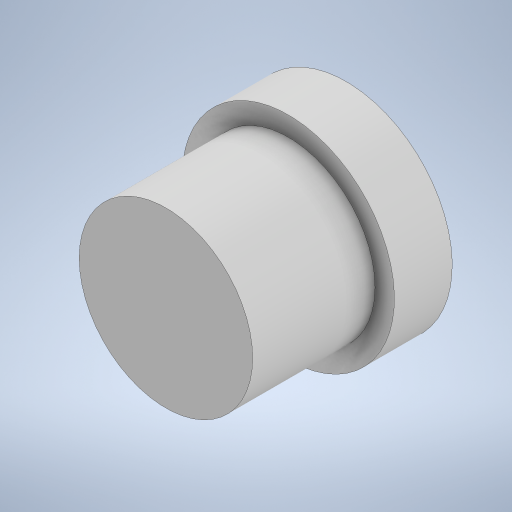
# Autodesk Inventor part: att_pin
Saved by Autodesk Inventor 2023.1 (Build 271208000, 208)
## iProperties
Created: 2024-12-03
Part Number: att_pin
Material: Типовые
Document SubType Name: Modeling
Designer: DELL
Density: 1 g/cm^3
Appearance: По умолчанию
Author: DELL
Autodesk Inventor part; units mm, degrees
(part 1 of 2)
ref_plane "YZ Plane" through (0, 0, 0) normal (1, 0, 0) x (0, 1, 0)
ref_plane "XZ Plane" through (0, 0, 0) normal (0, 1, 0) x (-1, 0, 0)
ref_plane "XY Plane" through (0, 0, 0) normal (0, 0, 1) x (1, 0, 0)
sketch "Эскиз1" plane through (0, 0, 0) normal (0, 0, 1) x (1, 0, 0)
  circle A0 centre (5.7181, 0.7273) radius 3.0026 construction
  ellipse E0 centre (5.709, 0.7156) end of major axis (2.2813, -3.5903) minor radius 5.5036 projected
  circle A1 centre (5.709, 0.7156) radius 2.75
  point P0 (0, 0)
  dimension "d4" = 5.5
  constraints: 1 centre point, 1 coincident, 1 other
  measures "d4" diameter of A1
extrude "Выдавливание1" add sketch "Эскиз1" along normal blind 3
sketch "Эскиз2" plane through (0, 0, 3) normal (0, 0, 1) x (1, 0, 0)
  spline S0 degree 3 poles (20.6934, -4.2961) (20.668, -4.2959) (20.6158, -4.2949) (20.5384, -4.2922) (20.4629, -4.2881) (20.3923, -4.2832) (20.3162, -4.2759) (20.2564, -4.2711) (20.212, -4.2637) (20.1912, -4.2611) (20.1707, -4.2589) (20.1505, -4.2572) (20.1304, -4.2562) (20.1104, -4.2558) (20.0904, -4.256) (20.0703, -4.2569) (20.0501, -4.2587) (20.0294, -4.2614) (20.0083, -4.2652) (19.9866, -4.2704) (19.964, -4.2773) (19.9404, -4.2862) (19.9158, -4.2978) (19.8904, -4.3128) (19.8644, -4.3319) (19.8387, -4.3557) (19.8146, -4.3847) (19.7945, -4.417) (19.7684, -4.4768) (19.7397, -4.5638) (19.7039, -4.6481) (19.6841, -4.7103) (19.6779, -4.7478) (19.6769, -4.7855) (19.6805, -4.8204) (19.6874, -4.8518) (19.6967, -4.8799) (19.7075, -4.9048) (19.7193, -4.9271) (19.7318, -4.9471) (19.7447, -4.9654) (19.7581, -4.9822) (19.7718, -4.9978) (19.7858, -5.0125) (19.8003, -5.0265) (19.8152, -5.0398) (19.8305, -5.0527) (19.8463, -5.0651) (19.8626, -5.0773) (19.8794, -5.0892) (19.8968, -5.1009) (19.9351, -5.1246) (19.9832, -5.1604) (20.0452, -5.2051) (20.1015, -5.248) (20.1609, -5.2947) (20.2209, -5.3437) (20.2608, -5.3774) (20.2801, -5.394) knots -0.738433 -0.738433 -0.738433 -0.738433 -0.721428 -0.703497 -0.686646 -0.670877 -0.656188 -0.635555 -0.630797 -0.626128 -0.621536 -0.617009 -0.612531 -0.608082 -0.603638 -0.599173 -0.594654 -0.590038 -0.585279 -0.580318 -0.575085 -0.569501 -0.563479 -0.55693 -0.549778 -0.541982 -0.533567 -0.524647 -0.516621 -0.490028 -0.463434 -0.455408 -0.446488 -0.438073 -0.430277 -0.423125 -0.416576 -0.410554 -0.40497 -0.399737 -0.394776 -0.390017 -0.385402 -0.380882 -0.376417 -0.371974 -0.367524 -0.363046 -0.358519 -0.353927 -0.349258 -0.3445 -0.323867 -0.309178 -0.293409 -0.276558 -0.258627 -0.241622 -0.241622 -0.241622 -0.241622 projected
  arc A0 (20.6934, -4.2961) -> (21.0569, -3.0396) centre (5.7104, 0.7186) ccw projected
  spline S1 degree 3 poles (21.2935, -1.8905) (21.2683, -1.8942) (21.2165, -1.9015) (21.1397, -1.9109) (21.0645, -1.9187) (20.994, -1.9249) (20.9177, -1.9295) (20.8579, -1.9342) (20.8129, -1.9338) (20.792, -1.9344) (20.7714, -1.9355) (20.7511, -1.937) (20.7311, -1.9392) (20.7112, -1.9419) (20.6915, -1.9452) (20.6719, -1.9493) (20.6521, -1.9542) (20.6322, -1.9601) (20.612, -1.9672) (20.5913, -1.9757) (20.57, -1.986) (20.5481, -1.9985) (20.5257, -2.0139) (20.5029, -2.0326) (20.4802, -2.0555) (20.4586, -2.0831) (20.4393, -2.1155) (20.4245, -2.1505) (20.408, -2.2137) (20.3933, -2.3041) (20.3711, -2.393) (20.3613, -2.4574) (20.361, -2.4955) (20.366, -2.5329) (20.375, -2.5668) (20.3867, -2.5967) (20.4003, -2.623) (20.4149, -2.6459) (20.43, -2.6661) (20.4455, -2.6839) (20.4611, -2.6999) (20.4769, -2.7144) (20.4929, -2.7277) (20.5091, -2.7401) (20.5255, -2.7516) (20.5423, -2.7624) (20.5595, -2.7727) (20.577, -2.7826) (20.595, -2.792) (20.6135, -2.8011) (20.6325, -2.81) (20.674, -2.8274) (20.7271, -2.8553) (20.7953, -2.8897) (20.8577, -2.9233) (20.9237, -2.9601) (20.9906, -2.9991) (21.0353, -3.0262) (21.0569, -3.0396) knots -0.738433 -0.738433 -0.738433 -0.738433 -0.721428 -0.703497 -0.686646 -0.670877 -0.656188 -0.635555 -0.630797 -0.626128 -0.621536 -0.617009 -0.612531 -0.608082 -0.603638 -0.599173 -0.594654 -0.590038 -0.585279 -0.580318 -0.575085 -0.569501 -0.563479 -0.55693 -0.549778 -0.541982 -0.533567 -0.524647 -0.516621 -0.490028 -0.463434 -0.455408 -0.446488 -0.438073 -0.430277 -0.423125 -0.416576 -0.410554 -0.40497 -0.399737 -0.394776 -0.390017 -0.385402 -0.380882 -0.376417 -0.371974 -0.367524 -0.363046 -0.358519 -0.353927 -0.349258 -0.3445 -0.323867 -0.309178 -0.293409 -0.276558 -0.258627 -0.241622 -0.241622 -0.241622 -0.241622 projected
  arc A1 (21.2935, -1.8905) -> (21.4559, -0.5926) centre (5.7104, 0.7186) ccw projected
  spline S2 degree 3 poles (21.5098, 0.5793) (21.4855, 0.5717) (21.4355, 0.5565) (21.3611, 0.5352) (21.288, 0.5157) (21.2193, 0.4986) (21.1448, 0.482) (21.0864, 0.4681) (21.0419, 0.4614) (21.0213, 0.4575) (21.0011, 0.4533) (20.9813, 0.4485) (20.9619, 0.4433) (20.9428, 0.4375) (20.9238, 0.4312) (20.905, 0.424) (20.8863, 0.4161) (20.8675, 0.4072) (20.8486, 0.397) (20.8295, 0.3853) (20.8102, 0.3719) (20.7905, 0.356) (20.7707, 0.3374) (20.7511, 0.3153) (20.7323, 0.2891) (20.7153, 0.2585) (20.7013, 0.2235) (20.6921, 0.1866) (20.6858, 0.1217) (20.6854, 0.03) (20.6774, -0.0612) (20.6777, -0.1264) (20.6835, -0.1641) (20.6942, -0.2002) (20.7084, -0.2323) (20.7247, -0.26) (20.7422, -0.2838) (20.7602, -0.3042) (20.7783, -0.3218) (20.7963, -0.337) (20.8143, -0.3503) (20.8322, -0.3622) (20.85, -0.3728) (20.8679, -0.3824) (20.886, -0.3912) (20.9043, -0.3994) (20.9228, -0.4069) (20.9417, -0.4138) (20.961, -0.4204) (20.9807, -0.4264) (21.0008, -0.4322) (21.0445, -0.4429) (21.1013, -0.4622) (21.1741, -0.4855) (21.2409, -0.5089) (21.3118, -0.5349) (21.384, -0.563) (21.4324, -0.5828) (21.4559, -0.5926) knots -0.738433 -0.738433 -0.738433 -0.738433 -0.721428 -0.703497 -0.686646 -0.670877 -0.656188 -0.635555 -0.630797 -0.626128 -0.621536 -0.617009 -0.612531 -0.608082 -0.603638 -0.599173 -0.594654 -0.590038 -0.585279 -0.580318 -0.575085 -0.569501 -0.563479 -0.55693 -0.549778 -0.541982 -0.533567 -0.524647 -0.516621 -0.490028 -0.463434 -0.455408 -0.446488 -0.438073 -0.430277 -0.423125 -0.416576 -0.410554 -0.40497 -0.399737 -0.394776 -0.390017 -0.385402 -0.380882 -0.376417 -0.371974 -0.367524 -0.363046 -0.358519 -0.353927 -0.349258 -0.3445 -0.323867 -0.309178 -0.293409 -0.276558 -0.258627 -0.241622 -0.241622 -0.241622 -0.241622 projected
  arc A2 (21.5098, 0.5793) -> (21.4671, 1.8867) centre (5.7104, 0.7186) ccw projected
  spline S3 degree 3 poles (21.337, 3.0526) (21.3143, 3.0413) (21.2673, 3.0184) (21.1971, 2.9857) (21.128, 2.9551) (21.0628, 2.9274) (20.9917, 2.8994) (20.9363, 2.8765) (20.8934, 2.8629) (20.8737, 2.8559) (20.8544, 2.8485) (20.8356, 2.8408) (20.8172, 2.8326) (20.7992, 2.8239) (20.7815, 2.8146) (20.764, 2.8046) (20.7468, 2.7939) (20.7297, 2.7821) (20.7126, 2.7691) (20.6955, 2.7546) (20.6785, 2.7382) (20.6616, 2.7196) (20.645, 2.6981) (20.6291, 2.6732) (20.6146, 2.6444) (20.6025, 2.6115) (20.5942, 2.5747) (20.5909, 2.5368) (20.5948, 2.4717) (20.6088, 2.3811) (20.6151, 2.2897) (20.6257, 2.2254) (20.6372, 2.1891) (20.6534, 2.1551) (20.6725, 2.1256) (20.6929, 2.1008) (20.7139, 2.08) (20.7349, 2.0627) (20.7555, 2.0482) (20.7757, 2.036) (20.7956, 2.0256) (20.8151, 2.0167) (20.8344, 2.009) (20.8536, 2.0023) (20.8728, 1.9964) (20.8921, 1.9913) (20.9116, 1.9867) (20.9313, 1.9828) (20.9514, 1.9794) (20.9718, 1.9765) (20.9926, 1.9739) (21.0374, 1.9702) (21.0966, 1.96) (21.1721, 1.9484) (21.2417, 1.9358) (21.3159, 1.9211) (21.3916, 1.9047) (21.4424, 1.8927) (21.4671, 1.8867) knots -0.738433 -0.738433 -0.738433 -0.738433 -0.721428 -0.703497 -0.686646 -0.670877 -0.656188 -0.635555 -0.630797 -0.626128 -0.621536 -0.617009 -0.612531 -0.608082 -0.603638 -0.599173 -0.594654 -0.590038 -0.585279 -0.580318 -0.575085 -0.569501 -0.563479 -0.55693 -0.549778 -0.541982 -0.533567 -0.524647 -0.516621 -0.490028 -0.463434 -0.455408 -0.446488 -0.438073 -0.430277 -0.423125 -0.416576 -0.410554 -0.40497 -0.399737 -0.394776 -0.390017 -0.385402 -0.380882 -0.376417 -0.371974 -0.367524 -0.363046 -0.358519 -0.353927 -0.349258 -0.3445 -0.323867 -0.309178 -0.293409 -0.276558 -0.258627 -0.241622 -0.241622 -0.241622 -0.241622 projected
  arc A3 (21.337, 3.0526) -> (21.0904, 4.3372) centre (5.7104, 0.7186) ccw projected
  spline S4 degree 3 poles (20.7795, 5.4684) (20.7588, 5.4537) (20.716, 5.4238) (20.6517, 5.3805) (20.5883, 5.3394) (20.5283, 5.3019) (20.4625, 5.2631) (20.4113, 5.2318) (20.371, 5.2117) (20.3526, 5.2016) (20.3347, 5.1913) (20.3174, 5.1807) (20.3005, 5.1698) (20.2841, 5.1584) (20.2681, 5.1464) (20.2524, 5.1339) (20.237, 5.1205) (20.2219, 5.1062) (20.2071, 5.0907) (20.1925, 5.0737) (20.1783, 5.0549) (20.1645, 5.0338) (20.1514, 5.01) (20.1396, 4.9829) (20.1298, 4.9522) (20.1231, 4.9178) (20.1206, 4.8802) (20.1233, 4.8422) (20.1373, 4.7785) (20.1653, 4.6913) (20.1858, 4.602) (20.2063, 4.5401) (20.2234, 4.506) (20.2448, 4.475) (20.2682, 4.4489) (20.2923, 4.4275) (20.3163, 4.4103) (20.3397, 4.3965) (20.3623, 4.3854) (20.3842, 4.3765) (20.4054, 4.3693) (20.426, 4.3636) (20.4463, 4.359) (20.4663, 4.3554) (20.4862, 4.3526) (20.5061, 4.3505) (20.5261, 4.3491) (20.5462, 4.3483) (20.5665, 4.3481) (20.5871, 4.3484) (20.6081, 4.3491) (20.6529, 4.3524) (20.7129, 4.3517) (20.7893, 4.352) (20.8601, 4.3504) (20.9356, 4.3475) (21.013, 4.3431) (21.0651, 4.3393) (21.0904, 4.3372) knots -0.738433 -0.738433 -0.738433 -0.738433 -0.721428 -0.703497 -0.686646 -0.670877 -0.656188 -0.635555 -0.630797 -0.626128 -0.621536 -0.617009 -0.612531 -0.608082 -0.603638 -0.599173 -0.594654 -0.590038 -0.585279 -0.580318 -0.575085 -0.569501 -0.563479 -0.55693 -0.549778 -0.541982 -0.533567 -0.524647 -0.516621 -0.490028 -0.463434 -0.455408 -0.446488 -0.438073 -0.430277 -0.423125 -0.416576 -0.410554 -0.40497 -0.399737 -0.394776 -0.390017 -0.385402 -0.380882 -0.376417 -0.371974 -0.367524 -0.363046 -0.358519 -0.353927 -0.349258 -0.3445 -0.323867 -0.309178 -0.293409 -0.276558 -0.258627 -0.241622 -0.241622 -0.241622 -0.241622 projected
  arc A4 (20.7795, 5.4684) -> (20.335, 6.6987) centre (5.7104, 0.7186) ccw projected
  spline S5 degree 3 poles (19.851, 7.7673) (19.8328, 7.7495) (19.7952, 7.7132) (19.7385, 7.6604) (19.6823, 7.6099) (19.6289, 7.5635) (19.5699, 7.5149) (19.5243, 7.4759) (19.4877, 7.4498) (19.4711, 7.437) (19.455, 7.424) (19.4395, 7.4108) (19.4246, 7.3974) (19.4101, 7.3835) (19.3962, 7.3692) (19.3827, 7.3544) (19.3696, 7.3388) (19.3569, 7.3223) (19.3447, 7.3047) (19.333, 7.2856) (19.3218, 7.2648) (19.3115, 7.2418) (19.3023, 7.2162) (19.2949, 7.1876) (19.29, 7.1558) (19.2887, 7.1208) (19.2921, 7.0832) (19.3008, 7.0461) (19.3246, 6.9854) (19.3658, 6.9036) (19.4001, 6.8187) (19.4301, 6.7607) (19.4522, 6.7298) (19.4782, 6.7024) (19.5054, 6.6803) (19.5325, 6.663) (19.5589, 6.6497) (19.5842, 6.6397) (19.6083, 6.6323) (19.6313, 6.6269) (19.6534, 6.6232) (19.6747, 6.6208) (19.6954, 6.6194) (19.7157, 6.619) (19.7358, 6.6193) (19.7558, 6.6204) (19.7757, 6.6221) (19.7957, 6.6245) (19.8158, 6.6274) (19.8361, 6.6309) (19.8567, 6.635) (19.9005, 6.6452) (19.9599, 6.6539) (20.0353, 6.6661) (20.1054, 6.6756) (20.1805, 6.6846) (20.2576, 6.6924) (20.3096, 6.6967) (20.335, 6.6987) knots -0.738433 -0.738433 -0.738433 -0.738433 -0.721428 -0.703497 -0.686646 -0.670877 -0.656188 -0.635555 -0.630797 -0.626128 -0.621536 -0.617009 -0.612531 -0.608082 -0.603638 -0.599173 -0.594654 -0.590038 -0.585279 -0.580318 -0.575085 -0.569501 -0.563479 -0.55693 -0.549778 -0.541982 -0.533567 -0.524647 -0.516621 -0.490028 -0.463434 -0.455408 -0.446488 -0.438073 -0.430277 -0.423125 -0.416576 -0.410554 -0.40497 -0.399737 -0.394776 -0.390017 -0.385402 -0.380882 -0.376417 -0.371974 -0.367524 -0.363046 -0.358519 -0.353927 -0.349258 -0.3445 -0.323867 -0.309178 -0.293409 -0.276558 -0.258627 -0.241622 -0.241622 -0.241622 -0.241622 projected
  arc A5 (19.851, 7.7673) -> (19.2195, 8.9128) centre (5.7104, 0.7186) ccw projected
  spline S6 degree 3 poles (18.5742, 9.8926) (18.5591, 9.8722) (18.5276, 9.8305) (18.4799, 9.7694) (18.4322, 9.7107) (18.3867, 9.6565) (18.3361, 9.5993) (18.2971, 9.5537) (18.2651, 9.5222) (18.2507, 9.5069) (18.2368, 9.4916) (18.2236, 9.4762) (18.2109, 9.4605) (18.1988, 9.4446) (18.1873, 9.4283) (18.1763, 9.4115) (18.1658, 9.3941) (18.1559, 9.3758) (18.1465, 9.3565) (18.1379, 9.3358) (18.1302, 9.3135) (18.1236, 9.2892) (18.1186, 9.2625) (18.1157, 9.2331) (18.1158, 9.2009) (18.12, 9.1661) (18.1293, 9.1295) (18.1436, 9.0942) (18.1766, 9.038) (18.2302, 8.9637) (18.2773, 8.8851) (18.316, 8.8326) (18.3427, 8.8054) (18.3726, 8.7825) (18.4029, 8.7649) (18.4325, 8.7521) (18.4606, 8.7431) (18.4871, 8.7372) (18.5121, 8.7336) (18.5356, 8.7319) (18.558, 8.7317) (18.5794, 8.7326) (18.6001, 8.7345) (18.6203, 8.7372) (18.6401, 8.7407) (18.6596, 8.7449) (18.679, 8.7497) (18.6984, 8.7552) (18.7178, 8.7612) (18.7373, 8.7679) (18.757, 8.7751) (18.7987, 8.7921) (18.856, 8.8099) (18.9285, 8.8338) (18.9963, 8.8542) (19.0691, 8.8748) (19.144, 8.8945) (19.1947, 8.907) (19.2195, 8.9128) knots -0.738433 -0.738433 -0.738433 -0.738433 -0.721428 -0.703497 -0.686646 -0.670877 -0.656188 -0.635555 -0.630797 -0.626128 -0.621536 -0.617009 -0.612531 -0.608082 -0.603638 -0.599173 -0.594654 -0.590038 -0.585279 -0.580318 -0.575085 -0.569501 -0.563479 -0.55693 -0.549778 -0.541982 -0.533567 -0.524647 -0.516621 -0.490028 -0.463434 -0.455408 -0.446488 -0.438073 -0.430277 -0.423125 -0.416576 -0.410554 -0.40497 -0.399737 -0.394776 -0.390017 -0.385402 -0.380882 -0.376417 -0.371974 -0.367524 -0.363046 -0.358519 -0.353927 -0.349258 -0.3445 -0.323867 -0.309178 -0.293409 -0.276558 -0.258627 -0.241622 -0.241622 -0.241622 -0.241622 projected
  arc A6 (18.5742, 9.8926) -> (17.7713, 10.9252) centre (5.7104, 0.7186) ccw projected
  spline S7 degree 3 poles (16.9807, 11.792) (16.969, 11.7694) (16.9444, 11.7233) (16.9068, 11.6556) (16.8689, 11.5902) (16.8325, 11.5295) (16.7914, 11.4651) (16.76, 11.4139) (16.7333, 11.3778) (16.7215, 11.3604) (16.7102, 11.3432) (16.6996, 11.3258) (16.6895, 11.3084) (16.68, 11.2908) (16.6712, 11.2729) (16.6629, 11.2546) (16.6553, 11.2357) (16.6484, 11.2161) (16.6422, 11.1956) (16.6369, 11.1738) (16.6327, 11.1506) (16.63, 11.1255) (16.6292, 11.0983) (16.631, 11.0689) (16.6362, 11.0371) (16.6458, 11.0034) (16.6606, 10.9687) (16.6803, 10.9361) (16.7217, 10.8857) (16.7862, 10.8207) (16.8451, 10.7505) (16.8915, 10.7046) (16.9221, 10.682) (16.9553, 10.664) (16.9879, 10.6514) (17.0191, 10.6433) (17.0483, 10.6389) (17.0755, 10.6372) (17.1007, 10.6376) (17.1242, 10.6396) (17.1463, 10.6428) (17.1673, 10.6471) (17.1875, 10.6522) (17.207, 10.6581) (17.226, 10.6646) (17.2446, 10.6718) (17.263, 10.6796) (17.2813, 10.688) (17.2995, 10.697) (17.3178, 10.7067) (17.3361, 10.7169) (17.3746, 10.7402) (17.4284, 10.7667) (17.4963, 10.8017) (17.5601, 10.8324) (17.6287, 10.8641) (17.6996, 10.8953) (17.7478, 10.9156) (17.7713, 10.9252) knots -0.738433 -0.738433 -0.738433 -0.738433 -0.721428 -0.703497 -0.686646 -0.670877 -0.656188 -0.635555 -0.630797 -0.626128 -0.621536 -0.617009 -0.612531 -0.608082 -0.603638 -0.599173 -0.594654 -0.590038 -0.585279 -0.580318 -0.575085 -0.569501 -0.563479 -0.55693 -0.549778 -0.541982 -0.533567 -0.524647 -0.516621 -0.490028 -0.463434 -0.455408 -0.446488 -0.438073 -0.430277 -0.423125 -0.416576 -0.410554 -0.40497 -0.399737 -0.394776 -0.390017 -0.385402 -0.380882 -0.376417 -0.371974 -0.367524 -0.363046 -0.358519 -0.353927 -0.349258 -0.3445 -0.323867 -0.309178 -0.293409 -0.276558 -0.258627 -0.241622 -0.241622 -0.241622 -0.241622 projected
  arc A7 (16.9807, 11.792) -> (16.0261, 12.6863) centre (5.7104, 0.7186) ccw projected
  spline S8 degree 3 poles (15.1097, 13.4187) (15.1016, 13.3946) (15.0846, 13.3452) (15.058, 13.2724) (15.0308, 13.2019) (15.0044, 13.1363) (14.9739, 13.0662) (14.9509, 13.0108) (14.9301, 12.9709) (14.9212, 12.9519) (14.9127, 12.9331) (14.9049, 12.9143) (14.8977, 12.8955) (14.8911, 12.8767) (14.8852, 12.8576) (14.8799, 12.8382) (14.8753, 12.8184) (14.8715, 12.7979) (14.8686, 12.7767) (14.8668, 12.7544) (14.8664, 12.7308) (14.8676, 12.7056) (14.8711, 12.6786) (14.8774, 12.6498) (14.8875, 12.6192) (14.9022, 12.5874) (14.9223, 12.5555) (14.9469, 12.5264) (14.9957, 12.4831) (15.0696, 12.4289) (15.1387, 12.3688) (15.1917, 12.3308) (15.2255, 12.3133) (15.261, 12.3007) (15.2953, 12.2933) (15.3273, 12.2902) (15.3569, 12.2904) (15.3839, 12.2929) (15.4088, 12.2973) (15.4317, 12.3029) (15.453, 12.3096) (15.4731, 12.3171) (15.4922, 12.3253) (15.5106, 12.3342) (15.5283, 12.3436) (15.5456, 12.3536) (15.5626, 12.3642) (15.5793, 12.3754) (15.5959, 12.3871) (15.6124, 12.3995) (15.6289, 12.4124) (15.6632, 12.4415) (15.7122, 12.4761) (15.7739, 12.5213) (15.832, 12.5616) (15.8949, 12.6036) (15.96, 12.6456) (16.0044, 12.6731) (16.0261, 12.6863) knots -0.738433 -0.738433 -0.738433 -0.738433 -0.721428 -0.703497 -0.686646 -0.670877 -0.656188 -0.635555 -0.630797 -0.626128 -0.621536 -0.617009 -0.612531 -0.608082 -0.603638 -0.599173 -0.594654 -0.590038 -0.585279 -0.580318 -0.575085 -0.569501 -0.563479 -0.55693 -0.549778 -0.541982 -0.533567 -0.524647 -0.516621 -0.490028 -0.463434 -0.455408 -0.446488 -0.438073 -0.430277 -0.423125 -0.416576 -0.410554 -0.40497 -0.399737 -0.394776 -0.390017 -0.385402 -0.380882 -0.376417 -0.371974 -0.367524 -0.363046 -0.358519 -0.353927 -0.349258 -0.3445 -0.323867 -0.309178 -0.293409 -0.276558 -0.258627 -0.241622 -0.241622 -0.241622 -0.241622 projected
  arc A8 (15.1097, 13.4187) -> (14.027, 14.1527) centre (5.7104, 0.7186) ccw projected
  spline S9 degree 3 poles (13.0073, 14.7327) (13.003, 14.7077) (12.9939, 14.6562) (12.9791, 14.5802) (12.9633, 14.5063) (12.9474, 14.4373) (12.9283, 14.3633) (12.9142, 14.305) (12.9, 14.2623) (12.8941, 14.2422) (12.8887, 14.2223) (12.8839, 14.2025) (12.8797, 14.1828) (12.8762, 14.1632) (12.8733, 14.1434) (12.8711, 14.1234) (12.8697, 14.1031) (12.8691, 14.0823) (12.8696, 14.0609) (12.8713, 14.0386) (12.8745, 14.0152) (12.8797, 13.9905) (12.8873, 13.9644) (12.8981, 13.9369) (12.9129, 13.9083) (12.9324, 13.8792) (12.9572, 13.8509) (12.986, 13.8259) (13.041, 13.7908) (13.1224, 13.7489) (13.2001, 13.7003) (13.2584, 13.671) (13.2945, 13.659) (13.3316, 13.6521) (13.3666, 13.6502) (13.3987, 13.6522) (13.4279, 13.6569) (13.4542, 13.6637) (13.4781, 13.6719) (13.4998, 13.6811) (13.5199, 13.691) (13.5385, 13.7016) (13.5561, 13.7126) (13.5728, 13.7242) (13.5889, 13.7363) (13.6044, 13.7489) (13.6195, 13.762) (13.6343, 13.7757) (13.6488, 13.7899) (13.6632, 13.8047) (13.6775, 13.8201) (13.7069, 13.8541) (13.7498, 13.896) (13.8036, 13.9502) (13.8548, 13.9991) (13.9102, 14.0505) (13.968, 14.1021) (14.0076, 14.1362) (14.027, 14.1527) knots -0.738433 -0.738433 -0.738433 -0.738433 -0.721428 -0.703497 -0.686646 -0.670877 -0.656188 -0.635555 -0.630797 -0.626128 -0.621536 -0.617009 -0.612531 -0.608082 -0.603638 -0.599173 -0.594654 -0.590038 -0.585279 -0.580318 -0.575085 -0.569501 -0.563479 -0.55693 -0.549778 -0.541982 -0.533567 -0.524647 -0.516621 -0.490028 -0.463434 -0.455408 -0.446488 -0.438073 -0.430277 -0.423125 -0.416576 -0.410554 -0.40497 -0.399737 -0.394776 -0.390017 -0.385402 -0.380882 -0.376417 -0.371974 -0.367524 -0.363046 -0.358519 -0.353927 -0.349258 -0.3445 -0.323867 -0.309178 -0.293409 -0.276558 -0.258627 -0.241622 -0.241622 -0.241622 -0.241622 projected
  arc A9 (13.0073, 14.7327) -> (11.823, 15.2883) centre (5.7104, 0.7186) ccw projected
  spline S10 degree 3 poles (10.7251, 15.7017) (10.7249, 15.6763) (10.7239, 15.624) (10.7212, 15.5466) (10.7171, 15.4711) (10.7122, 15.4005) (10.7049, 15.3245) (10.7001, 15.2646) (10.6927, 15.2203) (10.6901, 15.1995) (10.6879, 15.179) (10.6862, 15.1587) (10.6852, 15.1386) (10.6848, 15.1186) (10.685, 15.0986) (10.6859, 15.0786) (10.6877, 15.0583) (10.6904, 15.0377) (10.6942, 15.0166) (10.6994, 14.9948) (10.7063, 14.9722) (10.7152, 14.9487) (10.7269, 14.9241) (10.7418, 14.8986) (10.7609, 14.8726) (10.7847, 14.847) (10.8137, 14.8228) (10.846, 14.8027) (10.9058, 14.7766) (10.9928, 14.748) (11.0771, 14.7121) (11.1393, 14.6923) (11.1768, 14.6861) (11.2145, 14.6851) (11.2494, 14.6887) (11.2808, 14.6957) (11.3089, 14.7049) (11.3338, 14.7157) (11.3561, 14.7275) (11.3761, 14.74) (11.3944, 14.753) (11.4112, 14.7663) (11.4268, 14.78) (11.4415, 14.7941) (11.4555, 14.8085) (11.4688, 14.8234) (11.4817, 14.8387) (11.4941, 14.8545) (11.5063, 14.8708) (11.5182, 14.8877) (11.5299, 14.9051) (11.5536, 14.9433) (11.5895, 14.9914) (11.6341, 15.0534) (11.677, 15.1097) (11.7237, 15.1691) (11.7727, 15.2291) (11.8065, 15.269) (11.823, 15.2883) knots -0.738433 -0.738433 -0.738433 -0.738433 -0.721428 -0.703497 -0.686646 -0.670877 -0.656188 -0.635555 -0.630797 -0.626128 -0.621536 -0.617009 -0.612531 -0.608082 -0.603638 -0.599173 -0.594654 -0.590038 -0.585279 -0.580318 -0.575085 -0.569501 -0.563479 -0.55693 -0.549778 -0.541982 -0.533567 -0.524647 -0.516621 -0.490028 -0.463434 -0.455408 -0.446488 -0.438073 -0.430277 -0.423125 -0.416576 -0.410554 -0.40497 -0.399737 -0.394776 -0.390017 -0.385402 -0.380882 -0.376417 -0.371974 -0.367524 -0.363046 -0.358519 -0.353927 -0.349258 -0.3445 -0.323867 -0.309178 -0.293409 -0.276558 -0.258627 -0.241622 -0.241622 -0.241622 -0.241622 projected
  arc A10 (10.7251, 15.7017) -> (9.4686, 16.0652) centre (5.7104, 0.7186) ccw projected
  spline S11 degree 3 poles (8.3195, 16.3017) (8.3233, 16.2765) (8.3305, 16.2248) (8.3399, 16.1479) (8.3477, 16.0727) (8.3539, 16.0022) (8.3585, 15.926) (8.3632, 15.8661) (8.3628, 15.8212) (8.3635, 15.8002) (8.3645, 15.7796) (8.3661, 15.7593) (8.3682, 15.7393) (8.3709, 15.7195) (8.3742, 15.6998) (8.3783, 15.6801) (8.3832, 15.6604) (8.3891, 15.6404) (8.3962, 15.6202) (8.4047, 15.5995) (8.415, 15.5783) (8.4275, 15.5564) (8.4429, 15.5339) (8.4616, 15.5111) (8.4845, 15.4885) (8.5121, 15.4668) (8.5445, 15.4475) (8.5795, 15.4327) (8.6427, 15.4163) (8.7331, 15.4016) (8.822, 15.3794) (8.8865, 15.3695) (8.9245, 15.3693) (8.9619, 15.3742) (8.9958, 15.3832) (9.0257, 15.395) (9.052, 15.4085) (9.0749, 15.4231) (9.0951, 15.4383) (9.113, 15.4537) (9.129, 15.4694) (9.1435, 15.4852) (9.1567, 15.5011) (9.1691, 15.5173) (9.1806, 15.5338) (9.1914, 15.5506) (9.2018, 15.5677) (9.2116, 15.5853) (9.2211, 15.6033) (9.2301, 15.6218) (9.239, 15.6408) (9.2564, 15.6822) (9.2843, 15.7354) (9.3187, 15.8036) (9.3523, 15.8659) (9.3891, 15.9319) (9.4281, 15.9988) (9.4552, 16.0435) (9.4686, 16.0652) knots -0.738433 -0.738433 -0.738433 -0.738433 -0.721428 -0.703497 -0.686646 -0.670877 -0.656188 -0.635555 -0.630797 -0.626128 -0.621536 -0.617009 -0.612531 -0.608082 -0.603638 -0.599173 -0.594654 -0.590038 -0.585279 -0.580318 -0.575085 -0.569501 -0.563479 -0.55693 -0.549778 -0.541982 -0.533567 -0.524647 -0.516621 -0.490028 -0.463434 -0.455408 -0.446488 -0.438073 -0.430277 -0.423125 -0.416576 -0.410554 -0.40497 -0.399737 -0.394776 -0.390017 -0.385402 -0.380882 -0.376417 -0.371974 -0.367524 -0.363046 -0.358519 -0.353927 -0.349258 -0.3445 -0.323867 -0.309178 -0.293409 -0.276558 -0.258627 -0.241622 -0.241622 -0.241622 -0.241622 projected
  arc A11 (8.3195, 16.3017) -> (7.0216, 16.4641) centre (5.7104, 0.7186) ccw projected
  spline S12 degree 3 poles (5.8497, 16.518) (5.8573, 16.4937) (5.8725, 16.4438) (5.8938, 16.3693) (5.9133, 16.2962) (5.9305, 16.2276) (5.947, 16.153) (5.961, 16.0946) (5.9676, 16.0502) (5.9715, 16.0295) (5.9758, 16.0094) (5.9805, 15.9896) (5.9857, 15.9701) (5.9915, 15.951) (5.9979, 15.9321) (6.005, 15.9133) (6.0129, 15.8945) (6.0219, 15.8758) (6.032, 15.8569) (6.0437, 15.8378) (6.0572, 15.8184) (6.073, 15.7988) (6.0916, 15.779) (6.1137, 15.7594) (6.1399, 15.7406) (6.1705, 15.7235) (6.2055, 15.7095) (6.2424, 15.7004) (6.3073, 15.6941) (6.399, 15.6937) (6.4902, 15.6856) (6.5554, 15.686) (6.5931, 15.6917) (6.6292, 15.7024) (6.6613, 15.7166) (6.689, 15.7329) (6.7129, 15.7504) (6.7332, 15.7684) (6.7508, 15.7865) (6.766, 15.8046) (6.7793, 15.8225) (6.7912, 15.8404) (6.8018, 15.8583) (6.8115, 15.8762) (6.8203, 15.8942) (6.8284, 15.9125) (6.8359, 15.9311) (6.8428, 15.9499) (6.8494, 15.9692) (6.8554, 15.9889) (6.8612, 16.0091) (6.8719, 16.0527) (6.8912, 16.1096) (6.9145, 16.1823) (6.9379, 16.2491) (6.9639, 16.3201) (6.992, 16.3923) (7.0118, 16.4407) (7.0216, 16.4641) knots -0.738433 -0.738433 -0.738433 -0.738433 -0.721428 -0.703497 -0.686646 -0.670877 -0.656188 -0.635555 -0.630797 -0.626128 -0.621536 -0.617009 -0.612531 -0.608082 -0.603638 -0.599173 -0.594654 -0.590038 -0.585279 -0.580318 -0.575085 -0.569501 -0.563479 -0.55693 -0.549778 -0.541982 -0.533567 -0.524647 -0.516621 -0.490028 -0.463434 -0.455408 -0.446488 -0.438073 -0.430277 -0.423125 -0.416576 -0.410554 -0.40497 -0.399737 -0.394776 -0.390017 -0.385402 -0.380882 -0.376417 -0.371974 -0.367524 -0.363046 -0.358519 -0.353927 -0.349258 -0.3445 -0.323867 -0.309178 -0.293409 -0.276558 -0.258627 -0.241622 -0.241622 -0.241622 -0.241622 projected
  arc A12 (5.8497, 16.518) -> (4.5423, 16.4754) centre (5.7104, 0.7186) ccw projected
  spline S13 degree 3 poles (3.3764, 16.3453) (3.3877, 16.3225) (3.4106, 16.2755) (3.4433, 16.2053) (3.4739, 16.1362) (3.5016, 16.0711) (3.5296, 16) (3.5525, 15.9445) (3.5661, 15.9016) (3.5731, 15.8819) (3.5805, 15.8626) (3.5882, 15.8438) (3.5964, 15.8254) (3.6051, 15.8074) (3.6144, 15.7897) (3.6244, 15.7723) (3.6351, 15.755) (3.6469, 15.7379) (3.6599, 15.7208) (3.6744, 15.7038) (3.6908, 15.6868) (3.7094, 15.6698) (3.731, 15.6532) (3.7559, 15.6373) (3.7846, 15.6228) (3.8175, 15.6108) (3.8543, 15.6024) (3.8922, 15.5992) (3.9573, 15.6031) (4.0479, 15.617) (4.1393, 15.6234) (4.2036, 15.6339) (4.2399, 15.6455) (4.2739, 15.6617) (4.3034, 15.6807) (4.3282, 15.7012) (4.349, 15.7222) (4.3663, 15.7431) (4.3808, 15.7638) (4.393, 15.784) (4.4034, 15.8038) (4.4123, 15.8233) (4.42, 15.8426) (4.4267, 15.8618) (4.4326, 15.881) (4.4377, 15.9003) (4.4423, 15.9198) (4.4462, 15.9396) (4.4496, 15.9596) (4.4525, 15.98) (4.4551, 16.0008) (4.4588, 16.0457) (4.469, 16.1048) (4.4806, 16.1803) (4.4932, 16.2499) (4.5079, 16.3241) (4.5243, 16.3998) (4.5363, 16.4507) (4.5423, 16.4754) knots -0.738433 -0.738433 -0.738433 -0.738433 -0.721428 -0.703497 -0.686646 -0.670877 -0.656188 -0.635555 -0.630797 -0.626128 -0.621536 -0.617009 -0.612531 -0.608082 -0.603638 -0.599173 -0.594654 -0.590038 -0.585279 -0.580318 -0.575085 -0.569501 -0.563479 -0.55693 -0.549778 -0.541982 -0.533567 -0.524647 -0.516621 -0.490028 -0.463434 -0.455408 -0.446488 -0.438073 -0.430277 -0.423125 -0.416576 -0.410554 -0.40497 -0.399737 -0.394776 -0.390017 -0.385402 -0.380882 -0.376417 -0.371974 -0.367524 -0.363046 -0.358519 -0.353927 -0.349258 -0.3445 -0.323867 -0.309178 -0.293409 -0.276558 -0.258627 -0.241622 -0.241622 -0.241622 -0.241622 projected
  arc A13 (3.3764, 16.3453) -> (2.0918, 16.0987) centre (5.7104, 0.7186) ccw projected
  spline S14 degree 3 poles (0.9606, 15.7878) (0.9753, 15.7671) (1.0052, 15.7242) (1.0485, 15.66) (1.0896, 15.5965) (1.1272, 15.5365) (1.1659, 15.4707) (1.1972, 15.4195) (1.2173, 15.3793) (1.2274, 15.3609) (1.2377, 15.343) (1.2483, 15.3256) (1.2592, 15.3088) (1.2706, 15.2923) (1.2826, 15.2763) (1.2951, 15.2606) (1.3085, 15.2453) (1.3228, 15.2302) (1.3383, 15.2154) (1.3553, 15.2008) (1.3741, 15.1865) (1.3952, 15.1727) (1.419, 15.1597) (1.4461, 15.1479) (1.4768, 15.1381) (1.5112, 15.1313) (1.5488, 15.1288) (1.5868, 15.1315) (1.6505, 15.1456) (1.7377, 15.1735) (1.827, 15.1941) (1.8889, 15.2146) (1.923, 15.2317) (1.954, 15.253) (1.9801, 15.2764) (2.0015, 15.3005) (2.0187, 15.3245) (2.0325, 15.3479) (2.0436, 15.3705) (2.0525, 15.3924) (2.0597, 15.4136) (2.0654, 15.4343) (2.07, 15.4546) (2.0736, 15.4746) (2.0764, 15.4945) (2.0785, 15.5143) (2.0799, 15.5343) (2.0807, 15.5544) (2.0809, 15.5747) (2.0806, 15.5954) (2.0799, 15.6163) (2.0766, 15.6612) (2.0773, 15.7212) (2.077, 15.7976) (2.0786, 15.8683) (2.0815, 15.9439) (2.0859, 16.0212) (2.0897, 16.0733) (2.0918, 16.0987) knots -0.738433 -0.738433 -0.738433 -0.738433 -0.721428 -0.703497 -0.686646 -0.670877 -0.656188 -0.635555 -0.630797 -0.626128 -0.621536 -0.617009 -0.612531 -0.608082 -0.603638 -0.599173 -0.594654 -0.590038 -0.585279 -0.580318 -0.575085 -0.569501 -0.563479 -0.55693 -0.549778 -0.541982 -0.533567 -0.524647 -0.516621 -0.490028 -0.463434 -0.455408 -0.446488 -0.438073 -0.430277 -0.423125 -0.416576 -0.410554 -0.40497 -0.399737 -0.394776 -0.390017 -0.385402 -0.380882 -0.376417 -0.371974 -0.367524 -0.363046 -0.358519 -0.353927 -0.349258 -0.3445 -0.323867 -0.309178 -0.293409 -0.276558 -0.258627 -0.241622 -0.241622 -0.241622 -0.241622 projected
  arc A14 (0.9606, 15.7878) -> (-0.2696, 15.3432) centre (5.7104, 0.7186) ccw projected
  spline S15 degree 3 poles (-1.3383, 14.8592) (-1.3205, 14.8411) (-1.2842, 14.8034) (-1.2314, 14.7468) (-1.1809, 14.6905) (-1.1344, 14.6371) (-1.0859, 14.5782) (-1.0469, 14.5325) (-1.0208, 14.4959) (-1.008, 14.4793) (-0.995, 14.4633) (-0.9818, 14.4478) (-0.9684, 14.4328) (-0.9545, 14.4184) (-0.9402, 14.4044) (-0.9254, 14.3909) (-0.9098, 14.3778) (-0.8933, 14.3652) (-0.8757, 14.3529) (-0.8566, 14.3412) (-0.8358, 14.3301) (-0.8128, 14.3197) (-0.7872, 14.3106) (-0.7586, 14.3032) (-0.7268, 14.2983) (-0.6918, 14.297) (-0.6542, 14.3004) (-0.6171, 14.309) (-0.5564, 14.3328) (-0.4746, 14.3741) (-0.3896, 14.4084) (-0.3317, 14.4383) (-0.3007, 14.4605) (-0.2734, 14.4864) (-0.2513, 14.5136) (-0.234, 14.5408) (-0.2207, 14.5672) (-0.2107, 14.5924) (-0.2033, 14.6165) (-0.1979, 14.6395) (-0.1942, 14.6616) (-0.1918, 14.6829) (-0.1904, 14.7037) (-0.1899, 14.724) (-0.1903, 14.7441) (-0.1914, 14.764) (-0.1931, 14.784) (-0.1955, 14.8039) (-0.1984, 14.8241) (-0.2019, 14.8444) (-0.206, 14.865) (-0.2162, 14.9087) (-0.2249, 14.9681) (-0.2371, 15.0435) (-0.2466, 15.1137) (-0.2556, 15.1887) (-0.2634, 15.2658) (-0.2677, 15.3179) (-0.2696, 15.3432) knots -0.738433 -0.738433 -0.738433 -0.738433 -0.721428 -0.703497 -0.686646 -0.670877 -0.656188 -0.635555 -0.630797 -0.626128 -0.621536 -0.617009 -0.612531 -0.608082 -0.603638 -0.599173 -0.594654 -0.590038 -0.585279 -0.580318 -0.575085 -0.569501 -0.563479 -0.55693 -0.549778 -0.541982 -0.533567 -0.524647 -0.516621 -0.490028 -0.463434 -0.455408 -0.446488 -0.438073 -0.430277 -0.423125 -0.416576 -0.410554 -0.40497 -0.399737 -0.394776 -0.390017 -0.385402 -0.380882 -0.376417 -0.371974 -0.367524 -0.363046 -0.358519 -0.353927 -0.349258 -0.3445 -0.323867 -0.309178 -0.293409 -0.276558 -0.258627 -0.241622 -0.241622 -0.241622 -0.241622 projected
  arc A15 (-1.3383, 14.8592) -> (-2.4838, 14.2277) centre (5.7104, 0.7186) ccw projected
  spline S16 degree 3 poles (-3.4636, 13.5825) (-3.4431, 13.5673) (-3.4014, 13.5358) (-3.3404, 13.4881) (-3.2817, 13.4405) (-3.2275, 13.395) (-3.1703, 13.3444) (-3.1247, 13.3054) (-3.0931, 13.2733) (-3.0779, 13.2589) (-3.0626, 13.2451) (-3.0472, 13.2318) (-3.0315, 13.2192) (-3.0156, 13.2071) (-2.9993, 13.1955) (-2.9825, 13.1845) (-2.9651, 13.174) (-2.9468, 13.1641) (-2.9275, 13.1548) (-2.9068, 13.1462) (-2.8845, 13.1384) (-2.8602, 13.1318) (-2.8335, 13.1268) (-2.8041, 13.1239) (-2.7718, 13.1241) (-2.7371, 13.1283) (-2.7005, 13.1375) (-2.6652, 13.1519) (-2.609, 13.1849) (-2.5347, 13.2384) (-2.4561, 13.2856) (-2.4035, 13.3242) (-2.3764, 13.351) (-2.3535, 13.3809) (-2.3359, 13.4112) (-2.3231, 13.4407) (-2.3141, 13.4688) (-2.3082, 13.4954) (-2.3046, 13.5203) (-2.3029, 13.5439) (-2.3027, 13.5663) (-2.3036, 13.5877) (-2.3055, 13.6084) (-2.3082, 13.6285) (-2.3117, 13.6483) (-2.3159, 13.6679) (-2.3207, 13.6873) (-2.3262, 13.7067) (-2.3322, 13.7261) (-2.3389, 13.7456) (-2.3461, 13.7653) (-2.3631, 13.8069) (-2.3809, 13.8642) (-2.4048, 13.9368) (-2.4252, 14.0046) (-2.4458, 14.0773) (-2.4655, 14.1522) (-2.478, 14.203) (-2.4838, 14.2277) knots -0.738433 -0.738433 -0.738433 -0.738433 -0.721428 -0.703497 -0.686646 -0.670877 -0.656188 -0.635555 -0.630797 -0.626128 -0.621536 -0.617009 -0.612531 -0.608082 -0.603638 -0.599173 -0.594654 -0.590038 -0.585279 -0.580318 -0.575085 -0.569501 -0.563479 -0.55693 -0.549778 -0.541982 -0.533567 -0.524647 -0.516621 -0.490028 -0.463434 -0.455408 -0.446488 -0.438073 -0.430277 -0.423125 -0.416576 -0.410554 -0.40497 -0.399737 -0.394776 -0.390017 -0.385402 -0.380882 -0.376417 -0.371974 -0.367524 -0.363046 -0.358519 -0.353927 -0.349258 -0.3445 -0.323867 -0.309178 -0.293409 -0.276558 -0.258627 -0.241622 -0.241622 -0.241622 -0.241622 projected
  arc A16 (-3.4636, 13.5825) -> (-4.4962, 12.7795) centre (5.7104, 0.7186) ccw projected
  spline S17 degree 3 poles (-5.363, 11.989) (-5.3404, 11.9772) (-5.2943, 11.9526) (-5.2266, 11.915) (-5.1612, 11.8772) (-5.1005, 11.8407) (-5.0361, 11.7997) (-4.9849, 11.7683) (-4.9487, 11.7416) (-4.9314, 11.7297) (-4.9142, 11.7185) (-4.8968, 11.7078) (-4.8794, 11.6978) (-4.8618, 11.6883) (-4.8439, 11.6794) (-4.8256, 11.6712) (-4.8067, 11.6635) (-4.7871, 11.6566) (-4.7666, 11.6504) (-4.7448, 11.6451) (-4.7216, 11.641) (-4.6965, 11.6383) (-4.6693, 11.6375) (-4.6398, 11.6393) (-4.6081, 11.6444) (-4.5744, 11.654) (-4.5397, 11.6689) (-4.5071, 11.6885) (-4.4567, 11.73) (-4.3917, 11.7945) (-4.3215, 11.8533) (-4.2756, 11.8997) (-4.253, 11.9304) (-4.235, 11.9635) (-4.2224, 11.9962) (-4.2143, 12.0274) (-4.2099, 12.0566) (-4.2082, 12.0837) (-4.2086, 12.1089) (-4.2106, 12.1324) (-4.2138, 12.1546) (-4.2181, 12.1756) (-4.2232, 12.1957) (-4.2291, 12.2152) (-4.2356, 12.2342) (-4.2428, 12.2529) (-4.2506, 12.2713) (-4.259, 12.2896) (-4.268, 12.3078) (-4.2777, 12.326) (-4.2878, 12.3443) (-4.3111, 12.3828) (-4.3377, 12.4366) (-4.3727, 12.5046) (-4.4034, 12.5683) (-4.4351, 12.6369) (-4.4663, 12.7078) (-4.4866, 12.756) (-4.4962, 12.7795) knots -0.738433 -0.738433 -0.738433 -0.738433 -0.721428 -0.703497 -0.686646 -0.670877 -0.656188 -0.635555 -0.630797 -0.626128 -0.621536 -0.617009 -0.612531 -0.608082 -0.603638 -0.599173 -0.594654 -0.590038 -0.585279 -0.580318 -0.575085 -0.569501 -0.563479 -0.55693 -0.549778 -0.541982 -0.533567 -0.524647 -0.516621 -0.490028 -0.463434 -0.455408 -0.446488 -0.438073 -0.430277 -0.423125 -0.416576 -0.410554 -0.40497 -0.399737 -0.394776 -0.390017 -0.385402 -0.380882 -0.376417 -0.371974 -0.367524 -0.363046 -0.358519 -0.353927 -0.349258 -0.3445 -0.323867 -0.309178 -0.293409 -0.276558 -0.258627 -0.241622 -0.241622 -0.241622 -0.241622 projected
  arc A17 (-5.363, 11.989) -> (-6.2573, 11.0344) centre (5.7104, 0.7186) ccw projected
  spline S18 degree 3 poles (-6.9897, 10.118) (-6.9656, 10.1099) (-6.9162, 10.0928) (-6.8434, 10.0663) (-6.7729, 10.0391) (-6.7073, 10.0126) (-6.6372, 9.9821) (-6.5818, 9.9591) (-6.5419, 9.9384) (-6.5229, 9.9294) (-6.5041, 9.921) (-6.4853, 9.9132) (-6.4665, 9.906) (-6.4477, 9.8994) (-6.4286, 9.8934) (-6.4092, 9.8881) (-6.3894, 9.8836) (-6.3689, 9.8798) (-6.3477, 9.8769) (-6.3254, 9.8751) (-6.3018, 9.8746) (-6.2766, 9.8758) (-6.2496, 9.8793) (-6.2208, 9.8857) (-6.1902, 9.8958) (-6.1584, 9.9105) (-6.1265, 9.9306) (-6.0974, 9.9551) (-6.0541, 10.0039) (-5.9999, 10.0778) (-5.9398, 10.1469) (-5.9018, 10.1999) (-5.8842, 10.2337) (-5.8717, 10.2693) (-5.8643, 10.3035) (-5.8612, 10.3356) (-5.8614, 10.3651) (-5.8639, 10.3922) (-5.8683, 10.417) (-5.8739, 10.4399) (-5.8806, 10.4613) (-5.8881, 10.4814) (-5.8963, 10.5005) (-5.9052, 10.5188) (-5.9146, 10.5365) (-5.9246, 10.5538) (-5.9352, 10.5708) (-5.9464, 10.5875) (-5.9581, 10.6041) (-5.9705, 10.6206) (-5.9834, 10.6371) (-6.0124, 10.6715) (-6.0471, 10.7205) (-6.0923, 10.7821) (-6.1326, 10.8403) (-6.1746, 10.9031) (-6.2165, 10.9682) (-6.2441, 11.0127) (-6.2573, 11.0344) knots -0.738433 -0.738433 -0.738433 -0.738433 -0.721428 -0.703497 -0.686646 -0.670877 -0.656188 -0.635555 -0.630797 -0.626128 -0.621536 -0.617009 -0.612531 -0.608082 -0.603638 -0.599173 -0.594654 -0.590038 -0.585279 -0.580318 -0.575085 -0.569501 -0.563479 -0.55693 -0.549778 -0.541982 -0.533567 -0.524647 -0.516621 -0.490028 -0.463434 -0.455408 -0.446488 -0.438073 -0.430277 -0.423125 -0.416576 -0.410554 -0.40497 -0.399737 -0.394776 -0.390017 -0.385402 -0.380882 -0.376417 -0.371974 -0.367524 -0.363046 -0.358519 -0.353927 -0.349258 -0.3445 -0.323867 -0.309178 -0.293409 -0.276558 -0.258627 -0.241622 -0.241622 -0.241622 -0.241622 projected
  arc A18 (-6.9897, 10.118) -> (-7.7237, 9.0352) centre (5.7104, 0.7186) ccw projected
  spline S19 degree 3 poles (-8.3037, 8.0155) (-8.2787, 8.0113) (-8.2272, 8.0022) (-8.1512, 7.9873) (-8.0772, 7.9715) (-8.0083, 7.9556) (-7.9343, 7.9365) (-7.876, 7.9224) (-7.8333, 7.9082) (-7.8132, 7.9023) (-7.7933, 7.8969) (-7.7735, 7.8921) (-7.7538, 7.888) (-7.7342, 7.8844) (-7.7144, 7.8815) (-7.6944, 7.8793) (-7.6741, 7.8779) (-7.6533, 7.8774) (-7.6319, 7.8778) (-7.6096, 7.8795) (-7.5862, 7.8828) (-7.5615, 7.8879) (-7.5354, 7.8956) (-7.5079, 7.9064) (-7.4793, 7.9211) (-7.4502, 7.9406) (-7.4219, 7.9655) (-7.3969, 7.9943) (-7.3618, 8.0492) (-7.3199, 8.1307) (-7.2713, 8.2084) (-7.242, 8.2666) (-7.23, 8.3028) (-7.2231, 8.3398) (-7.2212, 8.3748) (-7.2232, 8.407) (-7.2279, 8.4361) (-7.2347, 8.4625) (-7.2429, 8.4863) (-7.2521, 8.5081) (-7.262, 8.5281) (-7.2725, 8.5468) (-7.2836, 8.5644) (-7.2952, 8.5811) (-7.3073, 8.5971) (-7.3199, 8.6126) (-7.333, 8.6277) (-7.3467, 8.6425) (-7.3609, 8.6571) (-7.3757, 8.6714) (-7.391, 8.6857) (-7.4251, 8.7151) (-7.467, 8.7581) (-7.5212, 8.8119) (-7.5701, 8.863) (-7.6215, 8.9185) (-7.6731, 8.9763) (-7.7072, 9.0158) (-7.7237, 9.0352) knots -0.738433 -0.738433 -0.738433 -0.738433 -0.721428 -0.703497 -0.686646 -0.670877 -0.656188 -0.635555 -0.630797 -0.626128 -0.621536 -0.617009 -0.612531 -0.608082 -0.603638 -0.599173 -0.594654 -0.590038 -0.585279 -0.580318 -0.575085 -0.569501 -0.563479 -0.55693 -0.549778 -0.541982 -0.533567 -0.524647 -0.516621 -0.490028 -0.463434 -0.455408 -0.446488 -0.438073 -0.430277 -0.423125 -0.416576 -0.410554 -0.40497 -0.399737 -0.394776 -0.390017 -0.385402 -0.380882 -0.376417 -0.371974 -0.367524 -0.363046 -0.358519 -0.353927 -0.349258 -0.3445 -0.323867 -0.309178 -0.293409 -0.276558 -0.258627 -0.241622 -0.241622 -0.241622 -0.241622 projected
  arc A19 (-8.3037, 8.0155) -> (-8.8593, 6.8313) centre (5.7104, 0.7186) ccw projected
  spline S20 degree 3 poles (-9.2727, 5.7334) (-9.2472, 5.7331) (-9.195, 5.7322) (-9.1176, 5.7294) (-9.0421, 5.7254) (-8.9715, 5.7205) (-8.8955, 5.7131) (-8.8356, 5.7084) (-8.7913, 5.701) (-8.7705, 5.6983) (-8.75, 5.6961) (-8.7297, 5.6945) (-8.7096, 5.6934) (-8.6896, 5.693) (-8.6696, 5.6932) (-8.6496, 5.6942) (-8.6293, 5.696) (-8.6087, 5.6987) (-8.5876, 5.7025) (-8.5658, 5.7077) (-8.5432, 5.7145) (-8.5196, 5.7235) (-8.4951, 5.7351) (-8.4696, 5.7501) (-8.4436, 5.7691) (-8.418, 5.793) (-8.3938, 5.8219) (-8.3737, 5.8543) (-8.3476, 5.914) (-8.3189, 6.001) (-8.2831, 6.0854) (-8.2633, 6.1475) (-8.2571, 6.1851) (-8.2561, 6.2228) (-8.2597, 6.2576) (-8.2667, 6.2891) (-8.2759, 6.3171) (-8.2867, 6.3421) (-8.2985, 6.3643) (-8.311, 6.3844) (-8.324, 6.4026) (-8.3373, 6.4194) (-8.351, 6.4351) (-8.3651, 6.4498) (-8.3795, 6.4637) (-8.3944, 6.4771) (-8.4097, 6.4899) (-8.4255, 6.5024) (-8.4418, 6.5145) (-8.4587, 6.5264) (-8.4761, 6.5381) (-8.5143, 6.5618) (-8.5624, 6.5977) (-8.6244, 6.6423) (-8.6807, 6.6852) (-8.7401, 6.732) (-8.8001, 6.781) (-8.84, 6.8147) (-8.8593, 6.8313) knots -0.738433 -0.738433 -0.738433 -0.738433 -0.721428 -0.703497 -0.686646 -0.670877 -0.656188 -0.635555 -0.630797 -0.626128 -0.621536 -0.617009 -0.612531 -0.608082 -0.603638 -0.599173 -0.594654 -0.590038 -0.585279 -0.580318 -0.575085 -0.569501 -0.563479 -0.55693 -0.549778 -0.541982 -0.533567 -0.524647 -0.516621 -0.490028 -0.463434 -0.455408 -0.446488 -0.438073 -0.430277 -0.423125 -0.416576 -0.410554 -0.40497 -0.399737 -0.394776 -0.390017 -0.385402 -0.380882 -0.376417 -0.371974 -0.367524 -0.363046 -0.358519 -0.353927 -0.349258 -0.3445 -0.323867 -0.309178 -0.293409 -0.276558 -0.258627 -0.241622 -0.241622 -0.241622 -0.241622 projected
  arc A20 (-9.2727, 5.7334) -> (-9.6362, 4.4768) centre (5.7104, 0.7186) ccw projected
  spline S21 degree 3 poles (-9.8727, 3.3278) (-9.8475, 3.3315) (-9.7958, 3.3387) (-9.7189, 3.3481) (-9.6437, 3.3559) (-9.5732, 3.3621) (-9.497, 3.3668) (-9.4371, 3.3715) (-9.3921, 3.3711) (-9.3712, 3.3717) (-9.3506, 3.3727) (-9.3303, 3.3743) (-9.3103, 3.3764) (-9.2905, 3.3791) (-9.2708, 3.3825) (-9.2511, 3.3865) (-9.2314, 3.3915) (-9.2114, 3.3974) (-9.1912, 3.4044) (-9.1705, 3.413) (-9.1493, 3.4233) (-9.1274, 3.4358) (-9.1049, 3.4511) (-9.0821, 3.4699) (-9.0594, 3.4928) (-9.0378, 3.5203) (-9.0185, 3.5527) (-9.0037, 3.5878) (-8.9873, 3.6509) (-8.9726, 3.7413) (-8.9504, 3.8302) (-8.9405, 3.8947) (-8.9403, 3.9328) (-8.9452, 3.9702) (-8.9542, 4.004) (-8.966, 4.034) (-8.9795, 4.0602) (-8.9941, 4.0832) (-9.0092, 4.1033) (-9.0247, 4.1212) (-9.0403, 4.1372) (-9.0561, 4.1517) (-9.0721, 4.165) (-9.0883, 4.1773) (-9.1048, 4.1888) (-9.1216, 4.1997) (-9.1387, 4.21) (-9.1562, 4.2198) (-9.1743, 4.2293) (-9.1928, 4.2384) (-9.2118, 4.2472) (-9.2532, 4.2646) (-9.3064, 4.2926) (-9.3746, 4.327) (-9.4369, 4.3605) (-9.5029, 4.3974) (-9.5698, 4.4364) (-9.6145, 4.4635) (-9.6362, 4.4768) knots -0.738433 -0.738433 -0.738433 -0.738433 -0.721428 -0.703497 -0.686646 -0.670877 -0.656188 -0.635555 -0.630797 -0.626128 -0.621536 -0.617009 -0.612531 -0.608082 -0.603638 -0.599173 -0.594654 -0.590038 -0.585279 -0.580318 -0.575085 -0.569501 -0.563479 -0.55693 -0.549778 -0.541982 -0.533567 -0.524647 -0.516621 -0.490028 -0.463434 -0.455408 -0.446488 -0.438073 -0.430277 -0.423125 -0.416576 -0.410554 -0.40497 -0.399737 -0.394776 -0.390017 -0.385402 -0.380882 -0.376417 -0.371974 -0.367524 -0.363046 -0.358519 -0.353927 -0.349258 -0.3445 -0.323867 -0.309178 -0.293409 -0.276558 -0.258627 -0.241622 -0.241622 -0.241622 -0.241622 projected
  arc A21 (-9.8727, 3.3278) -> (-10.0351, 2.0298) centre (5.7104, 0.7186) ccw projected
  spline S22 degree 3 poles (-10.089, 0.8579) (-10.0647, 0.8655) (-10.0148, 0.8808) (-9.9403, 0.9021) (-9.8672, 0.9216) (-9.7986, 0.9387) (-9.724, 0.9552) (-9.6656, 0.9692) (-9.6211, 0.9759) (-9.6005, 0.9798) (-9.5804, 0.984) (-9.5606, 0.9887) (-9.5411, 0.9939) (-9.522, 0.9997) (-9.5031, 1.0061) (-9.4843, 1.0132) (-9.4655, 1.0212) (-9.4468, 1.0301) (-9.4279, 1.0403) (-9.4088, 1.0519) (-9.3894, 1.0654) (-9.3698, 1.0812) (-9.35, 1.0999) (-9.3304, 1.122) (-9.3116, 1.1481) (-9.2945, 1.1787) (-9.2805, 1.2137) (-9.2714, 1.2507) (-9.265, 1.3156) (-9.2647, 1.4072) (-9.2566, 1.4985) (-9.257, 1.5637) (-9.2627, 1.6013) (-9.2734, 1.6375) (-9.2876, 1.6695) (-9.3039, 1.6973) (-9.3214, 1.7211) (-9.3394, 1.7415) (-9.3575, 1.759) (-9.3756, 1.7742) (-9.3935, 1.7876) (-9.4114, 1.7994) (-9.4293, 1.8101) (-9.4472, 1.8197) (-9.4652, 1.8285) (-9.4835, 1.8366) (-9.502, 1.8441) (-9.5209, 1.8511) (-9.5402, 1.8576) (-9.5599, 1.8637) (-9.5801, 1.8694) (-9.6237, 1.8802) (-9.6806, 1.8994) (-9.7533, 1.9227) (-9.8201, 1.9461) (-9.8911, 1.9722) (-9.9633, 2.0003) (-10.0117, 2.02) (-10.0351, 2.0298) knots -0.738433 -0.738433 -0.738433 -0.738433 -0.721428 -0.703497 -0.686646 -0.670877 -0.656188 -0.635555 -0.630797 -0.626128 -0.621536 -0.617009 -0.612531 -0.608082 -0.603638 -0.599173 -0.594654 -0.590038 -0.585279 -0.580318 -0.575085 -0.569501 -0.563479 -0.55693 -0.549778 -0.541982 -0.533567 -0.524647 -0.516621 -0.490028 -0.463434 -0.455408 -0.446488 -0.438073 -0.430277 -0.423125 -0.416576 -0.410554 -0.40497 -0.399737 -0.394776 -0.390017 -0.385402 -0.380882 -0.376417 -0.371974 -0.367524 -0.363046 -0.358519 -0.353927 -0.349258 -0.3445 -0.323867 -0.309178 -0.293409 -0.276558 -0.258627 -0.241622 -0.241622 -0.241622 -0.241622 projected
  arc A22 (-10.089, 0.8579) -> (-10.0464, -0.4495) centre (5.7104, 0.7186) ccw projected
  spline S23 degree 3 poles (-9.9163, -1.6154) (-9.8935, -1.604) (-9.8465, -1.5812) (-9.7763, -1.5485) (-9.7072, -1.5178) (-9.6421, -1.4901) (-9.571, -1.4621) (-9.5155, -1.4392) (-9.4726, -1.4257) (-9.4529, -1.4186) (-9.4336, -1.4113) (-9.4148, -1.4035) (-9.3964, -1.3953) (-9.3784, -1.3866) (-9.3607, -1.3773) (-9.3433, -1.3674) (-9.326, -1.3566) (-9.3089, -1.3448) (-9.2918, -1.3319) (-9.2748, -1.3174) (-9.2577, -1.301) (-9.2408, -1.2823) (-9.2242, -1.2608) (-9.2083, -1.2359) (-9.1938, -1.2071) (-9.1818, -1.1742) (-9.1734, -1.1375) (-9.1702, -1.0995) (-9.1741, -1.0344) (-9.188, -0.9439) (-9.1944, -0.8525) (-9.2049, -0.7881) (-9.2165, -0.7518) (-9.2327, -0.7178) (-9.2517, -0.6884) (-9.2722, -0.6635) (-9.2932, -0.6427) (-9.3141, -0.6254) (-9.3348, -0.6109) (-9.355, -0.5987) (-9.3748, -0.5883) (-9.3943, -0.5794) (-9.4136, -0.5717) (-9.4328, -0.565) (-9.452, -0.5592) (-9.4713, -0.554) (-9.4908, -0.5495) (-9.5106, -0.5456) (-9.5306, -0.5421) (-9.551, -0.5392) (-9.5718, -0.5367) (-9.6166, -0.5329) (-9.6758, -0.5228) (-9.7513, -0.5111) (-9.8209, -0.4985) (-9.8951, -0.4838) (-9.9708, -0.4674) (-10.0217, -0.4555) (-10.0464, -0.4495) knots -0.738433 -0.738433 -0.738433 -0.738433 -0.721428 -0.703497 -0.686646 -0.670877 -0.656188 -0.635555 -0.630797 -0.626128 -0.621536 -0.617009 -0.612531 -0.608082 -0.603638 -0.599173 -0.594654 -0.590038 -0.585279 -0.580318 -0.575085 -0.569501 -0.563479 -0.55693 -0.549778 -0.541982 -0.533567 -0.524647 -0.516621 -0.490028 -0.463434 -0.455408 -0.446488 -0.438073 -0.430277 -0.423125 -0.416576 -0.410554 -0.40497 -0.399737 -0.394776 -0.390017 -0.385402 -0.380882 -0.376417 -0.371974 -0.367524 -0.363046 -0.358519 -0.353927 -0.349258 -0.3445 -0.323867 -0.309178 -0.293409 -0.276558 -0.258627 -0.241622 -0.241622 -0.241622 -0.241622 projected
  arc A23 (-9.9163, -1.6154) -> (-9.6697, -2.9) centre (5.7104, 0.7186) ccw projected
  spline S24 degree 3 poles (-9.3588, -4.0312) (-9.338, -4.0164) (-9.2952, -3.9865) (-9.231, -3.9432) (-9.1675, -3.9021) (-9.1075, -3.8646) (-9.0417, -3.8258) (-8.9905, -3.7945) (-8.9503, -3.7744) (-8.9319, -3.7644) (-8.914, -3.7541) (-8.8966, -3.7435) (-8.8798, -3.7325) (-8.8633, -3.7211) (-8.8473, -3.7092) (-8.8316, -3.6966) (-8.8163, -3.6833) (-8.8012, -3.669) (-8.7864, -3.6535) (-8.7718, -3.6365) (-8.7575, -3.6177) (-8.7437, -3.5966) (-8.7307, -3.5727) (-8.7189, -3.5456) (-8.7091, -3.515) (-8.7023, -3.4806) (-8.6998, -3.443) (-8.7025, -3.405) (-8.7166, -3.3413) (-8.7445, -3.254) (-8.7651, -3.1648) (-8.7856, -3.1028) (-8.8026, -3.0688) (-8.824, -3.0377) (-8.8474, -3.0117) (-8.8715, -2.9903) (-8.8955, -2.9731) (-8.9189, -2.9592) (-8.9415, -2.9481) (-8.9634, -2.9392) (-8.9846, -2.9321) (-9.0053, -2.9263) (-9.0256, -2.9218) (-9.0456, -2.9181) (-9.0655, -2.9153) (-9.0853, -2.9133) (-9.1053, -2.9119) (-9.1254, -2.9111) (-9.1457, -2.9108) (-9.1664, -2.9111) (-9.1873, -2.9119) (-9.2322, -2.9152) (-9.2922, -2.9144) (-9.3686, -2.9147) (-9.4393, -2.9132) (-9.5149, -2.9103) (-9.5922, -2.9059) (-9.6443, -2.9021) (-9.6697, -2.9) knots -0.738433 -0.738433 -0.738433 -0.738433 -0.721428 -0.703497 -0.686646 -0.670877 -0.656188 -0.635555 -0.630797 -0.626128 -0.621536 -0.617009 -0.612531 -0.608082 -0.603638 -0.599173 -0.594654 -0.590038 -0.585279 -0.580318 -0.575085 -0.569501 -0.563479 -0.55693 -0.549778 -0.541982 -0.533567 -0.524647 -0.516621 -0.490028 -0.463434 -0.455408 -0.446488 -0.438073 -0.430277 -0.423125 -0.416576 -0.410554 -0.40497 -0.399737 -0.394776 -0.390017 -0.385402 -0.380882 -0.376417 -0.371974 -0.367524 -0.363046 -0.358519 -0.353927 -0.349258 -0.3445 -0.323867 -0.309178 -0.293409 -0.276558 -0.258627 -0.241622 -0.241622 -0.241622 -0.241622 projected
  arc A24 (-9.3588, -4.0312) -> (-8.9142, -5.2614) centre (5.7104, 0.7186) ccw projected
  spline S25 degree 3 poles (-8.4302, -6.33) (-8.412, -6.3122) (-8.3744, -6.276) (-8.3178, -6.2232) (-8.2615, -6.1727) (-8.2081, -6.1262) (-8.1492, -6.0776) (-8.1035, -6.0387) (-8.0669, -6.0125) (-8.0503, -5.9997) (-8.0342, -5.9868) (-8.0188, -5.9736) (-8.0038, -5.9601) (-7.9894, -5.9463) (-7.9754, -5.932) (-7.9619, -5.9171) (-7.9488, -5.9015) (-7.9361, -5.8851) (-7.9239, -5.8674) (-7.9122, -5.8484) (-7.9011, -5.8276) (-7.8907, -5.8046) (-7.8816, -5.779) (-7.8741, -5.7504) (-7.8693, -5.7185) (-7.868, -5.6835) (-7.8714, -5.646) (-7.88, -5.6089) (-7.9038, -5.5482) (-7.9451, -5.4664) (-7.9794, -5.3814) (-8.0093, -5.3235) (-8.0315, -5.2925) (-8.0574, -5.2652) (-8.0846, -5.2431) (-8.1118, -5.2257) (-8.1382, -5.2125) (-8.1634, -5.2025) (-8.1875, -5.1951) (-8.2105, -5.1897) (-8.2326, -5.1859) (-8.2539, -5.1835) (-8.2746, -5.1821) (-8.295, -5.1817) (-8.3151, -5.1821) (-8.335, -5.1831) (-8.3549, -5.1849) (-8.3749, -5.1872) (-8.3951, -5.1902) (-8.4154, -5.1937) (-8.436, -5.1977) (-8.4797, -5.208) (-8.5391, -5.2166) (-8.6145, -5.2289) (-8.6847, -5.2384) (-8.7597, -5.2474) (-8.8368, -5.2551) (-8.8889, -5.2595) (-8.9142, -5.2614) knots -0.738433 -0.738433 -0.738433 -0.738433 -0.721428 -0.703497 -0.686646 -0.670877 -0.656188 -0.635555 -0.630797 -0.626128 -0.621536 -0.617009 -0.612531 -0.608082 -0.603638 -0.599173 -0.594654 -0.590038 -0.585279 -0.580318 -0.575085 -0.569501 -0.563479 -0.55693 -0.549778 -0.541982 -0.533567 -0.524647 -0.516621 -0.490028 -0.463434 -0.455408 -0.446488 -0.438073 -0.430277 -0.423125 -0.416576 -0.410554 -0.40497 -0.399737 -0.394776 -0.390017 -0.385402 -0.380882 -0.376417 -0.371974 -0.367524 -0.363046 -0.358519 -0.353927 -0.349258 -0.3445 -0.323867 -0.309178 -0.293409 -0.276558 -0.258627 -0.241622 -0.241622 -0.241622 -0.241622 projected
  arc A25 (-8.4302, -6.33) -> (-7.7987, -7.4756) centre (5.7104, 0.7186) ccw projected